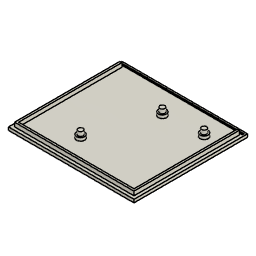
spodn kryt (Autodesk Fusion 360 design; units mm, degrees)
Autodesk Fusion 360 part; units mm, degrees
sketch "Sketch1" plane through (0, 0, 0) normal (0, 0, 1) x (1, 0, 0)
  circle A0 centre (69.6728, 78.3) radius 2.5
  circle A1 centre (10.1728, 16.1) radius 2.5
  line L0 (-29.7202, -5) -> (-29.7202, 96.8)
  line L1 (-29.7202, 96.8) -> (83.8798, 96.8)
  line L2 (83.8798, -5) -> (83.8798, 96.8)
  line L3 (-34.7202, -10) -> (88.8798, -10)
  line L4 (88.8798, -10) -> (88.8798, 96.8)
  line L5 (-34.7202, 96.8) -> (-34.7202, -10)
  line L6 (-31.7202, -7) -> (85.8798, -7)
  line L7 (85.8798, -7) -> (85.8798, 96.8)
  line L8 (-31.7202, 96.8) -> (-31.7202, -7)
  line L9 (-29.7202, -5) -> (83.8798, -5)
  circle A2 centre (10.1728, 16.1) radius 4
  circle A3 centre (31.1728, 75.7) radius 4
  circle A4 centre (69.6728, 78.3) radius 4
  circle A5 centre (31.1728, 75.7) radius 2.5
  line L10 (83.8798, 96.8) -> (88.8798, 96.8)
  line L11 (-29.7202, 96.8) -> (-34.7202, 96.8)
  dimension "d2" = 5
  dimension "d3" = 5
  dimension "d16" = 5
  dimension "d18" = 5
  dimension "d21" = 3
  dimension "d22" = 3
  dimension "d23" = 3
  dimension "d26" = 113.6
  dimension "d29" = 117.6
  dimension "d33" = 5
  dimension "d42" = 8
  dimension "d43" = 8
  dimension "d44" = 8
  dimension "d45" = 14.207
  dimension "d46" = 18.5
  dimension "d47" = 52.707
  dimension "d48" = 21.1
  dimension "d52" = 39.893
  dimension "d53" = 80.7
  dimension "d54" = 5
  dimension "d55" = 5
  constraint vertical L0
  constraint horizontal L1
  constraint vertical L2
  constraint horizontal L3
  constraint vertical L4
  constraint vertical L5
  constraint horizontal L6
  constraint vertical L7
  constraint vertical L8
  constraint horizontal L9
  constraint concentric A1 A2
  constraint concentric A0 A4
  constraint concentric A3 A5
  constraint perpendicular L4 L10
  constraint perpendicular L5 L11
  constraint coincident L11 L8.start
  constraint coincident L10 L7.end
  measures "d2" diameter of A0
  measures "d3" diameter of A1
  measures "d16" distance of L0 L5
  measures "d18" distance of L2 L4
  measures "d21" distance of L5 L8
  measures "d22" distance of L3 L6
  measures "d23" distance of L4 L7
  measures "d26" distance of L0.start L2.start
  measures "d29" distance of L6.start L6.end
  measures "d33" distance of L3 L9
  measures "d42" diameter of A2
  measures "d43" diameter of A3
  measures "d44" diameter of A4
  measures "d45" horizontal distance of A0.centre L1.end
  measures "d46" vertical distance of A0.centre L1.end
  measures "d47" horizontal distance of L1.end A3.centre
  measures "d48" vertical distance of L1.end A3.centre
  measures "d52" distance of A1.centre L0
  measures "d53" distance of A1.centre L1
  measures "d54" distance of origin L9
  measures "d55" diameter of A5
extrude "Extrude1" add sketch "Sketch1" along normal blind 3 contours L0 L1 L2 L9 | A2 | A3 | A4 | A5 makes body 1
extrude "Extrude2" add sketch "Sketch1" along normal blind 7 separate body contours L0 L2 L6 L7 L8 L9 L10 L11 makes body 2
extrude "Extrude3" add sketch "Sketch1" along normal blind 3 separate body contours L3 L4 L5 L6 L7 L8 L10 L11 makes body 3
extrude "Extrude4" add sketch "Sketch1" along normal blind 10 contours A0 | A1 bodies 1
extrude "Extrude5" add sketch "Sketch1" along normal blind 6 contours A2 | A3 | A4 | A5 bodies 1
extrude "Extrude6" add sketch "Sketch1" along normal blind 10 contours A5 bodies 1
sketch "Sketch2" plane through (88.8798, 0, 0) normal (1, 0, 0) x (0, 1, 0)
  line L0 (-10, 0) -> (96.8, 0)
  line L1 (96.8, 0) -> (96.8, 3)
  line L2 (96.8, 3) -> (-10, 3)
  line L3 (-10, 3) -> (-10, 0)
  line L4 (96.8, 0) -> (101.8, 0)
  line L5 (101.8, 0) -> (101.8, 3)
  line L6 (96.8, 3) -> (96.8, 0)
  line L7 (100.1, 3) -> (100.1, 1.7)
  line L8 (100.1, 1.7) -> (98.5, 1.7)
  line L9 (98.5, 1.7) -> (98.5, 3)
  line L10 (101.8, 3) -> (100.1, 3)
  line L11 (98.5, 3) -> (96.8, 3)
  dimension "d58" = 5
  dimension "d59" = 3
  dimension "d60" = 1.6
  dimension "d61" = 1.7
  dimension "d62" = 1.7
  constraint horizontal L4
  constraint vertical L5
  constraint horizontal L10
  constraint vertical L6
  constraint coincident L0.end L1.start
  constraint vertical L7
  constraint horizontal L8
  constraint vertical L9
  constraint coincident L9.end L10
  constraint collinear L10 L11
  measures "d58" distance of L0.end L4.end
  measures "d59" distance of L0.end L1.end
  measures "d60" distance of L7.end L8.end
  measures "d61" distance of L6 L9
  measures "d62" distance of L4 L8
extrude "Extrude7" add sketch "Sketch2" against normal blind 123.6 contours L1 L4 L5 L6 L7 L8 L9 L10 L11 bodies 1 2 3
sketch "Sketch3" plane through (0, 0, 3) normal (0, 0, 1) x (-1, 0, 0)
  line L0 (-85.8798, -96.8) -> (-85.8798, 7)
  line L1 (-85.8798, 7) -> (31.7202, 7)
  line L2 (31.7202, 7) -> (31.7202, -96.8)
  line L3 (31.7202, -96.8) -> (29.7202, -96.8)
  line L4 (29.7202, -96.8) -> (29.7202, 5)
  line L5 (29.7202, 5) -> (-83.8798, 5)
  line L6 (-83.8798, 5) -> (-83.8798, -96.8)
  line L7 (-83.8798, -96.8) -> (-85.8798, -96.8)
  circle A0 centre (-31.1728, -75.7) radius 4
  circle A1 centre (-10.1728, -16.1) radius 4
  circle A2 centre (-69.6728, -78.3) radius 4
  line L8 (-88.8798, 10) -> (-88.8798, -98.5)
  line L9 (-88.8798, -98.5) -> (34.7202, -98.5)
  line L10 (34.7202, -98.5) -> (34.7202, -96.8)
  line L11 (34.7202, -96.8) -> (34.7202, 10)
  line L12 (34.7202, 10) -> (-88.8798, 10)
  line L13 (34.7202, -98.5) -> (33.0202, -98.5)
  line L14 (33.0202, -98.5) -> (33.0202, -100.1)
  line L15 (33.0202, -100.1) -> (34.7202, -100.1)
  line L16 (34.7202, -100.1) -> (34.7202, -98.5)
  line L17 (-88.8798, -98.5) -> (-87.1798, -98.5)
  line L18 (-87.1798, -98.5) -> (-87.1798, -100.1)
  line L19 (-87.1798, -100.1) -> (-88.8798, -100.1)
  line L20 (-88.8798, -100.1) -> (-88.8798, -98.5)
  dimension "d65" = 1.7
  dimension "d66" = 1.6
  dimension "d67" = 1.7
  dimension "d68" = 1.6
  constraint horizontal L13
  constraint vertical L14
  constraint horizontal L15
  constraint vertical L16
  constraint coincident L9.end L10.start
  constraint horizontal L17
  constraint vertical L18
  constraint horizontal L19
  constraint vertical L20
  constraint coincident L8.end L9.start
  measures "d65" distance of L9.end L13.end
  measures "d66" distance of L9.end L15.end
  measures "d67" distance of L8.end L17.end
  measures "d68" distance of L8.end L19.end
extrude "Extrude8" add sketch "Sketch3" against normal blind 1.3 contours L9 L17 L18 L19 L20 | L9 L13 L14 L15 L16 bodies 1
